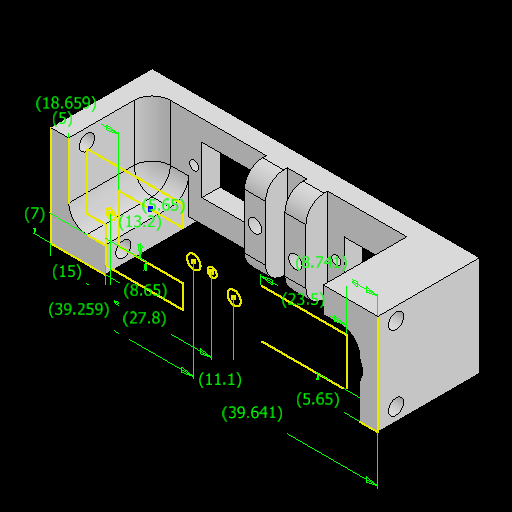
# Autodesk Inventor part: Frame
Saved by Autodesk Inventor 2023.2 (Build 272271030, 271C)
## iProperties
Created: 2023-11-22
Part Number: Frame
Material: Generic
Document SubType Name: Modeling
Designer: robpl
Density: 1 g/cm^3
Appearance: Default
Author: robpl
## iProperties of the stored document Frame_3DPrint.ipt
Created: 2023-11-27
Part Number: Frame_3DPrint
Material: Generic
Document SubType Name: Modeling
Designer: robpl
Density: 1 g/cm^3
Appearance: Default
Author: robpl
Autodesk Inventor part; units mm, degrees
ref_plane "YZ Plane" through (0, 0, 0) normal (1, 0, 0) x (0, 1, 0)
ref_plane "XZ Plane" through (0, 0, 0) normal (0, 1, 0) x (-1, 0, 0)
ref_plane "XY Plane" through (0, 0, 0) normal (0, 0, 1) x (1, 0, 0)
sketch "Sketch1" plane through (0, 0, 0) normal (0, 0, 1) x (1, 0, 0)
  line L0 (0, 0) -> (-90, 0)
  line L1 (-90, 0) -> (-90, -27.5)
  line L2 (-90, -27.5) -> (0, -27.5)
  line L3 (0, -27.5) -> (0, 0)
  line L4 (-90, 0) -> (-85, 0)
  line L5 (-85, 0) -> (-85, -20.5)
  line L6 (-85, -20.5) -> (-90, -20.5)
  line L7 (-90, -20.5) -> (-90, 0)
  line L8 (-90, -20.5) -> (-75, -20.5)
  line L9 (-75, -20.5) -> (-75, -27.5)
  line L10 (-75, -27.5) -> (-90, -27.5)
  line L11 (-90, -27.5) -> (-90, -20.5)
  line L12 (0, 0) -> (-15, 0)
  line L13 (-15, 0) -> (-15, -7)
  line L14 (-15, -7) -> (0, -7)
  line L15 (0, -7) -> (0, 0)
  line L16 (0, -27.5) -> (-5, -27.5)
  line L17 (-5, -27.5) -> (-5, -7)
  line L18 (-5, -7) -> (0, -7)
  line L19 (0, -7) -> (0, -27.5)
  dimension "d0" = 27.5
  dimension "d1" = 7
  dimension "d2" = 10
  dimension "d3" = 5
  dimension "d4" = 70
  constraints: 40 end point, 13 parallel, 5 horizontal, 5 perpendicular, 2 point on line
  measures "d0" distance between parallel lines of L0 L2
  measures "d1" distance of L12.end L13.end
  measures "d2" distance between parallel lines of L13 L17
  measures "d3" distance between parallel lines of L3 L17
  measures "d4" distance between parallel lines of L13 L5
extrude "Extrusion1" add sketch "Sketch1" along normal blind 10 contours L3 L14 L13 L0 | L3 L2 L17 L14 | L5 L6 L1 L0 | L8 L9 L2 L1 L6
sketch "Sketch2" plane through (0, -27.5, 0) normal (1, 0, 0) x (0, 0, -1)
  line L0 (0, 0) -> (0, 27.5) projected
  line L1 (0, 27.5) -> (-10, 27.5) projected
  line L2 (-10, 0) -> (-10, 27.5) projected
  line L3 (0, 0) -> (-10, 0) projected
  line L4 (-5, 3.525) -> (-5, 23.975)
  line L5 (-10, 20.5) -> (-10, 0) projected
  line L6 (-10, 0) -> (-10, 27.5)
  point P0 (-5, 0)
  point P1 (-10, 13.75)
  point P2 (-5, 13.75)
  dimension "d7" = 20.45
  dimension "d15" = 5
  constraints: 4 end point, 3 midpoint, 1 coincident, 1 collinear, 1 horizontal alignment, 1 vertical
  measures "d7" distance of L4.end point (-5, 3.525)
  measures "d15" distance between parallel lines of L2 L4
hole "Hole1" at (0, -3.525, 5) at (0, -23.975, 5) direction (-1, 0, 0) diameter 4.2 end through all
sketch "Sketch3" plane through (0, 0, 0) normal (0, 0, -1) x (-1, 0, 0)
  line L0 (75, -20.5) -> (85, -20.5) projected
  line L1 (75, -27.5) -> (75, -20.5) projected
  line L2 (90, -27.5) -> (75, -27.5) projected
  line L3 (90, 0) -> (90, -27.5) projected
  line L4 (85, 0) -> (90, 0) projected
  line L5 (85, -20.5) -> (85, 0) projected
  line L6 (5, -7) -> (5, -27.5) projected
  line L7 (15, -7) -> (5, -7) projected
  line L8 (15, 0) -> (15, -7) projected
  line L9 (0, 0) -> (15, 0) projected
  line L10 (0, -27.5) -> (0, 0) projected
  line L11 (5, -27.5) -> (0, -27.5) projected
  line L12 (5, -27.5) -> (0, -27.5) projected
  line L13 (0, -27.5) -> (0, 0) projected
  line L14 (5, -27.5) -> (0, -27.5)
  line L15 (0, -27.5) -> (0, 0)
  line L16 (0, 0) -> (5, 0)
  line L17 (5, 0) -> (5, -27.5)
  line L18 (85, 0) -> (90, 0)
  line L19 (90, 0) -> (90, -27.5)
  line L20 (90, -27.5) -> (85, -27.5)
  line L21 (85, -27.5) -> (85, 0)
  constraints: 16 end point, 4 parallel, 2 horizontal, 2 perpendicular
extrude "Extrusion2" add sketch "Sketch3" along normal blind 17.95
sketch "Sketch4" plane through (0, 0, -17.95) normal (0, 0, -1) x (-1, 0, 0)
  line L0 (75, -27.5) -> (90, -27.5) projected
  line L1 (90, -27.5) -> (90, 0) projected
  line L2 (90, 0) -> (85, 0) projected
  line L3 (85, 0) -> (85, -20.5) projected
  line L4 (15, 0) -> (0, 0) projected
  line L5 (0, 0) -> (0, -27.5) projected
  line L6 (0, -27.5) -> (5, -27.5) projected
  line L7 (5, -27.5) -> (5, -7) projected
  line L8 (5, 0) -> (15, 0) projected
  line L9 (85, -25.2) -> (85, -18.2) projected
  line L10 (5, 0) -> (85, 0)
  line L11 (85, 0) -> (85, -25.2)
  line L12 (85, -25.2) -> (5, -25.2)
  line L13 (5, -25.2) -> (5, 0)
  line L14 (75.6412, -7) -> (75.6412, -11.7) projected
  line L15 (74.4438, -11.7) -> (75.6412, -11.7) projected
  arc A0 (74.4438, -11.7) -> (74.4438, -12.8) centre (73.4912, -12.25) ccw projected
  line L16 (75.6412, -12.8) -> (74.4438, -12.8) projected
  line L17 (75.6412, -12.8) -> (75.6412, -17.5) projected
  arc A1 (74.7912, -18.35) -> (75.6412, -17.5) centre (74.7912, -17.5) ccw projected
  line L18 (74.7912, -18.35) -> (69.9912, -18.35) projected
  arc A2 (69.9912, -18.35) -> (70.8412, -17.5) centre (69.9912, -17.5) ccw projected
  line L19 (70.8412, -7) -> (70.8412, -17.5) projected
  arc A3 (70.8412, -7) -> (69.9912, -6.15) centre (69.9912, -7) ccw projected
  line L20 (69.9912, -6.15) -> (74.7912, -6.15) projected
  arc A4 (75.6412, -7) -> (74.7912, -6.15) centre (74.7912, -7) ccw projected
  arc A5 (44.7386, -12.8) -> (44.7386, -11.7) centre (45.6912, -12.25) ccw projected
  line L21 (43.5412, -11.7) -> (44.7386, -11.7) projected
  line L22 (43.5412, -11.7) -> (43.5412, -7) projected
  arc A6 (44.3912, -6.15) -> (43.5412, -7) centre (44.3912, -7) ccw projected
  line L23 (44.3912, -6.15) -> (49.1912, -6.15) projected
  arc A7 (49.1912, -6.15) -> (48.3412, -7) centre (49.1912, -7) ccw projected
  line L24 (48.3412, -17.5) -> (48.3412, -7) projected
  arc A8 (48.3412, -17.5) -> (49.1912, -18.35) centre (49.1912, -17.5) ccw projected
  line L25 (49.1912, -18.35) -> (44.3912, -18.35) projected
  arc A9 (43.5412, -17.5) -> (44.3912, -18.35) centre (44.3912, -17.5) ccw projected
  line L26 (43.5412, -17.5) -> (43.5412, -12.8) projected
  line L27 (44.7386, -12.8) -> (43.5412, -12.8) projected
  line L28 (36.5412, -10) -> (36.5412, -14.7) projected
  line L29 (35.3438, -14.7) -> (36.5412, -14.7) projected
  arc A10 (35.3438, -14.7) -> (35.3438, -15.8) centre (34.3912, -15.25) ccw projected
  line L30 (36.5412, -15.8) -> (35.3438, -15.8) projected
  line L31 (36.5412, -15.8) -> (36.5412, -20.5) projected
  arc A11 (35.6912, -21.35) -> (36.5412, -20.5) centre (35.6912, -20.5) ccw projected
  line L32 (35.6912, -21.35) -> (30.8912, -21.35) projected
  arc A12 (30.8912, -21.35) -> (31.7412, -20.5) centre (30.8912, -20.5) ccw projected
  line L33 (31.7412, -10) -> (31.7412, -20.5) projected
  arc A13 (31.7412, -10) -> (30.8912, -9.15) centre (30.8912, -10) ccw projected
  line L34 (30.8912, -9.15) -> (35.6912, -9.15) projected
  arc A14 (36.5412, -10) -> (35.6912, -9.15) centre (35.6912, -10) ccw projected
  arc A15 (5.6386, -15.8) -> (5.6386, -14.7) centre (6.5912, -15.25) ccw projected
  line L35 (4.4412, -14.7) -> (5.6386, -14.7) projected
  line L36 (4.4412, -14.7) -> (4.4412, -10) projected
  arc A16 (5.2912, -9.15) -> (4.4412, -10) centre (5.2912, -10) ccw projected
  line L37 (5.2912, -9.15) -> (10.0912, -9.15) projected
  arc A17 (10.0912, -9.15) -> (9.2412, -10) centre (10.0912, -10) ccw projected
  line L38 (9.2412, -20.5) -> (9.2412, -10) projected
  arc A18 (9.2412, -20.5) -> (10.0912, -21.35) centre (10.0912, -20.5) ccw projected
  line L39 (10.0912, -21.35) -> (5.2912, -21.35) projected
  arc A19 (4.4412, -20.5) -> (5.2912, -21.35) centre (5.2912, -20.5) ccw projected
  line L40 (4.4412, -20.5) -> (4.4412, -15.8) projected
  line L41 (5.6386, -15.8) -> (4.4412, -15.8) projected
  line L42 (9.2412, -9.15) -> (31.7412, -9.15)
  line L43 (31.7412, -9.15) -> (31.7412, -21.35)
  line L44 (31.7412, -21.35) -> (9.2412, -21.35)
  line L45 (9.2412, -21.35) -> (9.2412, -9.15)
  line L46 (48.3412, -6.15) -> (70.8412, -6.15)
  line L47 (70.8412, -6.15) -> (70.8412, -18.35)
  line L48 (70.8412, -18.35) -> (48.3412, -18.35)
  line L49 (48.3412, -18.35) -> (48.3412, -6.15)
  line L50 (8.7412, -8.65) -> (32.2412, -8.65)
  line L51 (32.2412, -8.65) -> (32.2412, -21.85)
  line L52 (32.2412, -21.85) -> (8.7412, -21.85)
  line L53 (8.7412, -21.85) -> (8.7412, -8.65)
  line L54 (47.8412, -5.65) -> (71.3412, -5.65)
  line L55 (71.3412, -5.65) -> (71.3412, -18.85)
  line L56 (71.3412, -18.85) -> (47.8412, -18.85)
  line L57 (47.8412, -18.85) -> (47.8412, -5.65)
  circle A20 centre (6.5912, -15.25) radius 1.25
  circle A21 centre (34.3912, -15.25) radius 1.25
  circle A22 centre (45.6912, -12.25) radius 1.25
  circle A23 centre (73.4912, -12.25) radius 1.25
  line L58 (5, -7) -> (15, -7) projected
  line L59 (15, -7) -> (15, 0) projected
  line L60 (85, -20.5) -> (75, -20.5) projected
  line L61 (75, -20.5) -> (75, -27.5) projected
  point P0 (75, -25.2)
  dimension "d18" = 0.5
  dimension "d19" = 0.5
  dimension "d20" = 2.5
  constraints: 40 end point, 10 parallel, 8 collinear, 5 perpendicular, 4 centre point, 4 coincident, 3 equal radius, 3 horizontal, 6 other
  measures "d18" distance between parallel lines of L45 L53
  measures "d19" distance between parallel lines of L49 L57
  measures "d20" diameter of A20
extrude "Extrusion3" add sketch "Sketch4" against normal blind 5 contours L12 L7 A19 L39 L53 L52 L51 L32 A11 L31 L30 A21 L29 L28 A14 L34 L50 L37 A16 L58 L59 L10 L3 L60 L61 | L7 L41 A20 L35 A16 L37 L53 L39 A19 | L7 L35 A20 L41 | L51 L34 A14 L28 L29 A21 L30 L31 A11 L32 | L14 L15 A23 L16 L17 A1 L18 L55 L20 A4 | L57 L25 A9 L26 L27 A22 L21 L22 A6 L23
sketch "Sketch5" plane through (0, 0, -12.95) normal (0, 0, 1) x (1, 0, 0)
  circle A0 centre (-50.7412, -12.25) radius 1.25 projected
  circle A1 centre (-39.6412, -15.25) radius 1.25 projected
  circle A2 centre (-6.5912, -15.25) radius 1.25 projected
  line L0 (-5, -7) -> (-5, -25.2) projected
  line L1 (-85, -20.5) -> (-85, 0) projected
  line L2 (-75, -25.2) -> (-5, -25.2) projected
  circle A3 centre (-73.4912, -12.25) radius 1.25 projected
  line L3 (-71.3412, -18.85) -> (-71.3412, -5.65) projected
  line L4 (-71.3412, -5.65) -> (-47.8412, -5.65) projected
  line L5 (-47.8412, -5.65) -> (-47.8412, -18.85) projected
  line L6 (-47.8412, -18.85) -> (-71.3412, -18.85) projected
  circle A4 centre (-45.6912, -12.25) radius 1.25 projected
  circle A5 centre (-34.3912, -15.25) radius 1.25 projected
  line L7 (-8.7412, -8.65) -> (-8.7412, -21.85) projected
  line L8 (-8.7412, -21.85) -> (-32.2412, -21.85) projected
  line L9 (-32.2412, -21.85) -> (-32.2412, -8.65) projected
  line L10 (-32.2412, -8.65) -> (-8.7412, -8.65) projected
  line L11 (-5, 0) -> (-85, 0) projected
  line L12 (-53.6412, 0) -> (-47.8412, 0)
  line L13 (-47.8412, 0) -> (-47.8412, -25.2)
  line L14 (-47.8412, -25.2) -> (-53.6412, -25.2)
  line L15 (-53.6412, -25.2) -> (-53.6412, 0)
  line L16 (-47.8412, -5.65) -> (-47.8412, -18.85) projected
  line L17 (-90, 0) -> (0, 0) projected
  line L18 (-42.5412, 0) -> (-36.7412, 0)
  line L19 (-36.7412, 0) -> (-36.7412, -25.2)
  line L20 (-36.7412, -25.2) -> (-42.5412, -25.2)
  line L21 (-42.5412, -25.2) -> (-42.5412, 0)
  line L22 (-75, -25.2) -> (-5, -25.2) projected
  line L23 (-75, -20.5) -> (-85, -20.5) projected
  line L24 (-75, -25.2) -> (-75, -20.5) projected
  line L25 (-15, -7) -> (-5, -7) projected
  line L26 (-15, 0) -> (-15, -7) projected
  line L27 (-15, 0) -> (-85, 0) projected
  point P0 (-85, -25.2)
  point P1 (-50.7412, 0)
  point P2 (-39.6412, -25.2)
  dimension "d23" = 5.8
  dimension "d24" = 5.8
  constraints: 16 end point, 4 parallel, 3 point on line, 2 collinear, 2 horizontal, 2 midpoint, 2 perpendicular, 2 vertical alignment
  measures "d23" distance between parallel lines of L15 L13
  measures "d24" distance between parallel lines of L19 L21
extrude "Extrusion4" add sketch "Sketch5" along normal blind 6 contours L2 L21 L11 L19 | L2 L15 L6 L13 | L6 L15 L4 L5 | L13 L4 L15 L11
sketch "Sketch6" plane through (0, 0, -6.95) normal (0, 0, 1) x (1, 0, 0)
  circle A0 centre (-50.7412, -12.25) radius 1.25 projected
  circle A1 centre (-39.6412, -15.25) radius 1.25 projected
  point P0 (0, 0)
hole "Hole2" at (-50.7412, -12.25, -6.95) at (-39.6412, -15.25, -6.95) direction (0, 0, -1) diameter 2.5 end through all counterbore diameter 3.7 counterbore depth 3.5
sketch "Sketch7" plane through (0, 0, -12.95) normal (0, 0, 1) x (1, 0, 0)
  circle A0 centre (-6.5912, -15.25) radius 1.25 projected
  circle A1 centre (-6.5912, -15.25) radius 2.5
  point P0 (0, 0)
  dimension "d34" = 5
  constraints: 1 centre point, 1 coincident
  measures "d34" diameter of A1
extrude "Extrusion5" cut sketch "Sketch7" along normal through all contours A0 | A1
fillet "Fillet1" radius 5 11 edges at (-5, -13.3218, -1.475) (-5, -17.1782, -1.475) (-85, -20.5, -1.475) (-50.7412, -25.2, -6.95) (-50.7412, 0, -6.95) (-39.6412, 0, -6.95) (-39.6412, -25.2, -6.95) (-85, -10.25, -12.95) (-80, -20.5, -12.95) (-5, -21.1891, -12.95) (-5, -7, -1.475)
sketch "Sketch8" plane through (0, 0, 10) normal (0, 0, 1) x (1, 0, 0)
  line L0 (-75, -25.2) -> (-75, -15.5) projected
  line L1 (-75, -25.2) -> (-53.6412, -25.2) projected
  line L2 (-53.6412, -25.2) -> (-53.6412, -18.85) projected
  line L3 (-53.6412, -18.85) -> (-71.3412, -18.85) projected
  line L4 (-71.3412, -18.85) -> (-71.3412, -5.65) projected
  line L5 (-71.3412, -5.65) -> (-53.6412, -5.65) projected
  line L6 (-53.6412, -5.65) -> (-53.6412, 0) projected
  line L7 (-53.6412, 0) -> (-80, 0) projected
  line L8 (-80, -15.5) -> (-80, 0) projected
  line L9 (-75, -15.5) -> (-80, -15.5) projected
  circle A0 centre (-73.4912, -12.25) radius 1.25 projected
  line L10 (-90, -27.5) -> (-75, -27.5) projected
  line L11 (-32.2412, -8.65) -> (-8.7412, -8.65) projected
  line L12 (-90, 0) -> (-90, -27.5) projected
  line L13 (0, -27.5) -> (0, 0) projected
  line L14 (-8.7412, -8.65) -> (-8.7412, -21.4205) projected
  line L15 (-5, -27.5) -> (0, -27.5) projected
  line L16 (-9.6841, -21.85) -> (-32.2412, -21.85) projected
  line L17 (-85, -15.5) -> (-85, 0) projected
  line L18 (-75, -20.5) -> (-80, -20.5) projected
  circle A1 centre (-45.6912, -12.25) radius 1.25 projected
  circle A2 centre (-39.6412, -15.25) radius 1.85 projected
  circle A3 centre (-50.7412, -12.25) radius 1.85 projected
  point P0 (-62.4912, -5.65)
  dimension "d38" = 5.65
  dimension "d39" = 13.2
  dimension "d40" = 8.65
  dimension "d41" = 23.5
  dimension "d42" = 18.6588
  dimension "d43" = 8.7412
  dimension "d44" = 5.65
  dimension "d45" = 5
  dimension "d46" = 15
  dimension "d47" = 7
  dimension "d48" = 27.8
  dimension "d49" = 11.1
  dimension "d50" = 39.2588
  dimension "d51" = 39.6412
  constraints: 1 midpoint
  measures "d38" distance from line of point (-62.491, -5.65) L7
  measures "d39" distance between parallel lines of L3 L5
  measures "d40" distance between parallel lines of L10 L3
  measures "d41" distance of L11.start L11.end
  measures "d42" distance between parallel lines of L12 L4
  measures "d43" distance between parallel lines of L13 L14
  measures "d44" distance between parallel lines of L15 L16
  measures "d45" distance between parallel lines of L12 L17
  measures "d46" distance between parallel lines of L12 L0
  measures "d47" distance between parallel lines of L10 L18
  measures "d48" distance of A0.centre A1.centre
  measures "d49" horizontal distance of A2.centre A3.centre
  measures "d50" distance from line of L12 A3.centre
  measures "d51" distance from line of L13 A2.centre
equation "\"d24\" = d23"
body "Solid1"
